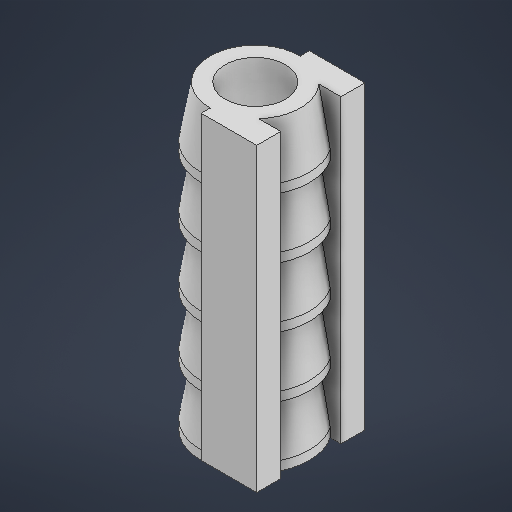
# Autodesk Inventor part: nipple
Saved by Autodesk Inventor 2026.2 (Build 302298000, 298)
## iProperties
Created: 2026-01-17
Part Number: nipple
Material: Generic
Document SubType Name: Modeling
Designer: User
Density: 1 g/cm^3
Appearance: Default
Author: User
Autodesk Inventor part; units mm, degrees
ref_plane "YZ Plane" through (0, 0, 0) normal (1, 0, 0) x (0, 1, 0)
ref_plane "XZ Plane" through (0, 0, 0) normal (0, 1, 0) x (-1, 0, 0)
ref_plane "XY Plane" through (0, 0, 0) normal (0, 0, 1) x (1, 0, 0)
sketch "Sketch1" plane through (0, 0, 0) normal (1, 0, 0) x (0, 1, 0)
  line L0 (0, -2) -> (4, -2)
  line L1 (4, -2) -> (4, -3)
  line L2 (4, -3) -> (0.5972, -3.6)
  line L3 (0, -3.6) -> (0, -2)
  line L4 (-4, 0) -> (24, 0) projected
  line L5 (0, -3.6) -> (0.5972, -3.6)
  line L6 (4, -2) -> (8, -2)
  line L7 (8, -2) -> (8, -3)
  line L8 (8, -3) -> (4.5972, -3.6)
  line L9 (4, -3.6) -> (4, -2)
  line L10 (4, -3.6) -> (4.5972, -3.6)
  line L11 (8, -2) -> (12, -2)
  line L12 (12, -2) -> (12, -3)
  line L13 (12, -3) -> (8.5972, -3.6)
  line L14 (8, -3.6) -> (8, -2)
  line L15 (8, -3.6) -> (8.5972, -3.6)
  line L16 (12, -2) -> (16, -2)
  line L17 (16, -2) -> (16, -3)
  line L18 (16, -3) -> (12.5972, -3.6)
  line L19 (12, -3.6) -> (12, -2)
  line L20 (12, -3.6) -> (12.5972, -3.6)
  line L21 (16, -2) -> (20, -2)
  line L22 (20, -2) -> (20, -3)
  line L23 (20, -3) -> (16.5972, -3.6)
  line L24 (16, -3.6) -> (16, -2)
  line L25 (16, -3.6) -> (16.5972, -3.6)
  point P0 (0, 0)
  dimension "d0" = 1
  dimension "d1" = 2
  dimension "d2" = 4
  dimension "d3" = 10
  dimension "d4" = 0
  dimension "d12" = 3.6
  dimension "d15" = 4
  constraints: 50 end point, 3 horizontal, 1 collinear, 1 parallel, 1 perpendicular, 39 other
  measures "d0" distance of L0.end L1.end
  measures "d1" distance between parallel lines of L4 L0
  measures "d2" distance of L0.start L0.end
  measures "d3" angle of L0 L2
  measures "d4" distance from line of point (0, 0) L3
  measures "d12" distance between parallel lines of L5 L4
  measures "d15" distance of L0.start L6.start
revolve "Revolution1" add sketch "Sketch1" angle 360 about axis through (0, -10, 0) along (0, 1, 0)
sketch "Sketch2" plane through (0, 0, 0) normal (1, 0, 0) x (0, 1, 0)
  line L0 (0, -3.6) -> (0, 3.6) projected
  line L1 (20, -2) -> (20, 2) projected
  line L2 (0, -3.6) -> (20, -3.6)
  line L3 (20, -3.6) -> (20, -2)
  line L4 (20, -2) -> (0, -2)
  line L5 (0, -2) -> (0, -3.6)
  line L6 (0, 3.6) -> (20, 3.6)
  line L7 (20, 3.6) -> (20, 2)
  line L8 (20, 2) -> (0, 2)
  line L9 (0, 2) -> (0, 3.6)
  point P0 (0, 0)
  point P1 (0, 1.6227)
  point P2 (20, -3.8756)
  dimension "d24" = 1.6
  constraints: 16 end point, 4 parallel, 2 horizontal, 2 perpendicular, 2 point on line
  measures "d24" distance of L6.end L7.end
extrude "Extrusion1" add sketch "Sketch2" along normal blind 3.7 contours L0 L4 L3 L2 | L0 L6 L7 L8
body "Solid1"
